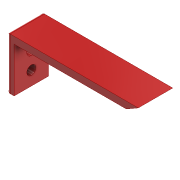
# Autodesk Inventor part: capstone ear
Saved by Autodesk Inventor 2020 (Build 240168000, 168)
## iProperties
Created: 2020-02-10
Part Number: capstone ear
Material: Generic
Document SubType Name: Modeling
Designer: ball
Density: 1 g/cm^3
Appearance: Default
Author: ball
Autodesk Inventor part; units mm, degrees
ref_plane "YZ Plane" through (0, 0, 0) normal (1, 0, 0) x (0, 1, 0)
ref_plane "XZ Plane" through (0, 0, 0) normal (0, 1, 0) x (-1, 0, 0)
ref_plane "XY Plane" through (0, 0, 0) normal (0, 0, 1) x (1, 0, 0)
sketch "Sketch1" plane through (0, 0, 0) normal (0, 1, 0) x (-1, 0, 0)
  line L0 (0, 6.35) -> (-45.72, 6.35)
  line L1 (-45.72, 6.35) -> (-45.72, -6.35)
  line L2 (-45.72, -6.35) -> (0, -6.35)
  line L3 (0, -6.35) -> (0, 6.35)
  point P0 (0, 0)
  dimension "d0" = 45.72
  dimension "d1" = 12.7
  dimension "d2" = 6.35
  constraints: 8 end point, 2 parallel, 1 horizontal, 1 perpendicular
  measures "d0" distance of L2.end L1.end
  measures "d1" distance of L1.end L0.end
  measures "d2" distance from line of point (0, 0) L0
extrude "Extrusion1" add sketch "Sketch1" along normal blind 2.54
sketch "Sketch2" plane through (0, 2.54, 0) normal (0, 1, 0) x (1, 0, 0)
  line L0 (0, 6.35) -> (0, -6.35) projected
  line L1 (0, 6.35) -> (-2.54, 6.35)
  line L2 (-2.54, 6.35) -> (-2.54, -6.35)
  line L3 (-2.54, -6.35) -> (0, -6.35)
  line L4 (0, -6.35) -> (0, 6.35)
  point P0 (0, 0)
  point P1 (0, -6.35)
  dimension "d5" = 2.54
  constraints: 8 end point, 2 parallel, 1 horizontal, 1 perpendicular
  measures "d5" distance of L3.end L2.end
extrude "Extrusion2" add sketch "Sketch2" against normal blind 19.05
sketch "Sketch3" plane through (0, -16.51, 6.35) normal (1, 0, 0) x (0, 0, -1)
  circle A0 centre (6.35, 11.43) radius 1.7
  circle A1 centre (6.35, 5.08) radius 1.7
  line L0 (12.7, 16.51) -> (0, 16.51) projected
  point P0 (6.35, 16.51)
  dimension "d8" = 3.4
  dimension "d9" = 3.4
  dimension "d10" = 5.08
  dimension "d11" = 6.35
  constraints: 2 centre point
  measures "d8" diameter of A0
  measures "d9" diameter of A1
  measures "d10" distance from line of L0 A0.centre
  measures "d11" distance of A1.centre A0.centre
extrude "Extrusion3" cut sketch "Sketch3" against normal through all
fillet "Fillet1" radius 1.016 2 edges at (-2.54, 2.54, 0) (-2.54, -16.51, 0)
sketch "Sketch4" plane through (45.72, 0, 6.35) normal (0, 0, 1) x (1, 0, 0)
  line L0 (0, 0) -> (0, 2.54) projected
  line L1 (0, 2.54) -> (-4.3994, 0)
  line L2 (-45.72, 0) -> (0, 0) projected
  line L3 (0, 2.54) -> (5.08, 2.54) construction
  line L4 (-4.3994, 0) -> (0, 0)
  line L5 (0, 0) -> (0, 2.54)
  dimension "d15" = 150
  constraints: 8 end point, 2 horizontal, 1 equal length, 1 perpendicular, 1 point on line
  measures "d15" angle of L1 L3
extrude "Extrusion4" cut sketch "Sketch4" against normal through all
equation "\"d2\" = 0.5 * d1"
body "Solid1"
